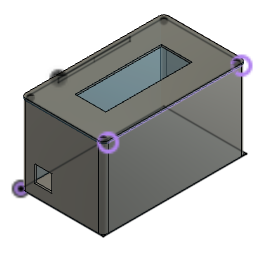
arduino_LED (Autodesk Fusion 360 design; units mm, degrees)
Autodesk Fusion 360 part; units mm, degrees
sketch "Base" plane through (0, 0, 0) normal (0, 1, 0) x (1, 0, 0) in component "Case"
  line L0 (0, 0) -> (68, 0)
  line L1 (68, 0) -> (68, 118)
  line L2 (68, 118) -> (0, 118)
  line L3 (0, 118) -> (0, 0)
  dimension "d6" = 68
  dimension "d7" = 118
  constraint horizontal L0
  constraint vertical L1
  constraint horizontal L2
  constraint vertical L3
  constraint coincident L0.start L3.end
  measures "d6" distance of L0.start L0.end
  measures "d7" distance of L0.start L2.end
extrude "Extrude1" add sketch "Base" along normal blind 65 makes body 1 in component "Case"
fillet "Fillet1" radius 4 4 edges at (68, 32.5, 0) (0, 32.5, 0) (68, 32.5, -118) (0, 32.5, -118) on bodies 1 in component "Case"
shell "Shell1" thickness 1.5 removed faces 1 at (22.6667, 65, -40.6667) on bodies 1 in component "Case"
sketch "Knob" plane through (1.5, 0, 0) normal (1, 0, 0) x (0, 0, -1) in component "Case"
  line L0 (114, 1.5) -> (114, 65)
  line L1 (114, 65) -> (4, 65)
  line L2 (4, 65) -> (4, 1.5)
  line L3 (4, 1.5) -> (114, 1.5)
  line L4 (29.5, 65) -> (88.5, 65)
  line L5 (88.5, 65) -> (88.5, 62)
  line L6 (88.5, 62) -> (29.5, 62)
  line L7 (29.5, 62) -> (29.5, 65)
  line L8 (59, 65) -> (59, 62) construction
  dimension "d12" = 59
  dimension "d13" = 3
  constraint horizontal L4
  constraint vertical L5
  constraint horizontal L6
  constraint vertical L7
  constraint coincident L1 L4.start
  constraint midpoint L1 L8.start
  constraint midpoint L6 L8.end
  constraint vertical L8
  measures "d12" distance of L5.end L6.end
  measures "d13" distance of L4.end L5.end
extrude "Extrude2" add sketch "Knob" along normal blind 6 draft -45 contours L1 L4 L5 L6 L7 bodies 1 in component "Case"
ref_plane "WorkPlane2" through (34, 32.5, -59) normal (-1, 0, 0) x (0, 0, 1) in component "Case"
mirror "Mirror1" about plane through (34, 32.5, -59) normal (-1, 0, 0) of "Extrude2" in component "Case"
sketch "Top" plane through (0, 65, 0) normal (0, 1, 0) x (-1, 0, 0) in component "Top Cover"
  line L0 (-68, -4) -> (-68, -114)
  arc A0 (-68, -114) -> (-64, -118) centre (-64, -114) ccw
  line L1 (-64, -118) -> (-4, -118)
  arc A1 (-4, -118) -> (0, -114) centre (-4, -114) ccw
  line L2 (0, -114) -> (0, -4)
  arc A2 (0, -4) -> (-4, 0) centre (-4, -4) ccw
  line L3 (-4, 0) -> (-64, 0)
  arc A3 (-64, 0) -> (-68, -4) centre (-64, -4) ccw
  line L4 (-66.5, -29.5) -> (-66.5, -4)
  arc A4 (-64, -1.5) -> (-66.5, -4) centre (-64, -4) ccw
  line L5 (-64, -1.5) -> (-4, -1.5)
  arc A5 (-1.5, -4) -> (-4, -1.5) centre (-4, -4) ccw
  line L6 (-1.5, -4) -> (-1.5, -29.5)
  line L7 (-1.5, -29.5) -> (-1.5, -88.5)
  line L8 (-1.5, -88.5) -> (-1.5, -114)
  arc A6 (-4, -116.5) -> (-1.5, -114) centre (-4, -114) ccw
  line L9 (-4, -116.5) -> (-64, -116.5)
  arc A7 (-66.5, -114) -> (-64, -116.5) centre (-64, -114) ccw
  line L10 (-66.5, -114) -> (-66.5, -88.5)
  line L11 (-66.5, -88.5) -> (-66.5, -29.5)
extrude "Extrude1'" add sketch "Top" along normal blind 1.5 separate body contours L0 A0 L1 A1 L2 A2 L3 A3 | L4 A4 L5 A5 L6 L7 L8 A6 L9 A7 L10 L11 makes body 2 in component "Top Cover"
sketch "Lip" plane through (0, 65, 0) normal (0, -1, 0) x (1, 0, 0) in component "Top Cover"
  arc A0 (68, -4) -> (64, 0) centre (64, -4) ccw
  line L0 (64, 0) -> (4, 0)
  arc A1 (4, 0) -> (0, -4) centre (4, -4) ccw
  line L1 (0, -4) -> (0, -114)
  arc A2 (0, -114) -> (4, -118) centre (4, -114) ccw
  line L2 (4, -118) -> (64, -118)
  arc A3 (64, -118) -> (68, -114) centre (64, -114) ccw
  line L3 (68, -114) -> (68, -4)
  line L4 (66.3, -114) -> (66.3, -4)
  arc A4 (66.3, -4) -> (64, -1.7) centre (64, -4) ccw
  line L5 (64, -1.7) -> (4, -1.7)
  arc A5 (4, -1.7) -> (1.7, -4) centre (4, -4) ccw
  line L6 (1.7, -4) -> (1.7, -114)
  arc A6 (1.7, -114) -> (4, -116.3) centre (4, -114) ccw
  line L7 (4, -116.3) -> (64, -116.3)
  arc A7 (64, -116.3) -> (66.3, -114) centre (64, -114) ccw
  line L8 (68, -4) -> (68, -114)
  dimension "d19" = 1.7
  dimension "d31" = 1.7
  measures "d31" distance of L4 L8
extrude "Extrude2'" add sketch "Lip" along normal blind 3 contours L4 A4 L5 A5 L6 A6 L7 A7 bodies 2 in component "Top Cover"
extrude "Extrude3" cut sketch "Knob" along normal blind 3 draft -45 from surface at 0.2 contours L1 L4 L5 L6 L7 bodies 2 in component "Top Cover"
ref_plane "WorkPlane2" through (34, 0, 0) normal (1, 0, 0) x (0, 1, 0) in component "Top Cover"
mirror "Mirror1'" about plane through (34, 0, 0) normal (1, 0, 0) of "Extrude3" in component "Top Cover"
shell "Shell1'" thickness 1.5 removed faces 1 at (44.7667, 62, -68.8333) on bodies 2 in component "Top Cover"
chamfer "Chamfer1" distance 0.6 angle 45 2 edges at (1.7, 62, -59) (66.3, 62, -59) on bodies 2 in component "Top Cover"
sketch "Sketch1" plane through (2.1865, 66.5, -5.8403) normal (0, 1, 0) x (-1, 0, 0)
  line L0 (-65.8135, 1.8403) -> (-65.8135, -108.1597)
  arc A0 (-65.8135, -108.1597) -> (-61.8135, -112.1597) centre (-61.8135, -108.1597) ccw
  line L1 (-61.8135, -112.1597) -> (-1.8135, -112.1597)
  arc A1 (-1.8135, -112.1597) -> (2.1865, -108.1597) centre (-1.8135, -108.1597) ccw
  line L2 (2.1865, -108.1597) -> (2.1865, 1.8403)
  arc A2 (2.1865, 1.8403) -> (-1.8135, 5.8403) centre (-1.8135, 1.8403) ccw
  line L3 (-1.8135, 5.8403) -> (-61.8135, 5.8403)
  arc A3 (-61.8135, 5.8403) -> (-65.8135, 1.8403) centre (-61.8135, 1.8403) ccw
  line L4 (-19.2135, -17.5597) -> (-44.4135, -17.5597)
  line L5 (-44.4135, -17.5597) -> (-44.4135, -88.7597)
  line L6 (-44.4135, -88.7597) -> (-19.2135, -88.7597)
  line L7 (-19.2135, -88.7597) -> (-19.2135, -17.5597)
  line L8 (2.1865, 5.8403) -> (-65.8135, 5.8403)
  line L9 (2.1865, -112.1597) -> (2.1865, 5.8403)
  dimension "d36" = 25.2
  dimension "d37" = 71.2
  dimension "d38" = 23.4
  dimension "d39" = 21.4
  constraint horizontal L4
  constraint vertical L5
  constraint horizontal L6
  constraint vertical L7
  measures "d36" distance of L4.start L4.end
  measures "d37" distance of L4.start L6.end
  measures "d38" distance of L4 L8
  measures "d39" distance of L7 L9
extrude "Extrude4" cut sketch "Sketch1" against normal blind 2 contours L4 L5 L6 L7 bodies 2 in component "Top Cover"
sketch "Sketch2" plane through (0, 0, 0) normal (0, 0, 1) x (1, 0, 0)
  line L0 (4, 65) -> (4, 0)
  line L1 (4, 0) -> (64, 0)
  line L2 (64, 0) -> (64, 65)
  line L3 (64, 65) -> (4, 65)
  line L4 (11.5, 23.5) -> (25.5, 23.5)
  line L5 (25.5, 23.5) -> (25.5, 9.5)
  line L6 (25.5, 9.5) -> (11.5, 9.5)
  line L7 (11.5, 9.5) -> (11.5, 23.5)
  line L8 (0, 65) -> (0, 0)
  line L9 (0, 0) -> (68, 0)
  dimension "d42" = 14
  dimension "d43" = 14
  dimension "d44" = 11.5
  dimension "d45" = 9.5
  constraint horizontal L4
  constraint vertical L5
  constraint horizontal L6
  constraint vertical L7
  measures "d42" distance of L4.start L4.end
  measures "d43" distance of L4.start L6.end
  measures "d44" distance of L7 L8
  measures "d45" distance of L6 L9
extrude "Extrude3'" cut sketch "Sketch2" against normal blind 2 contours L4 L5 L6 L7 bodies 1 in component "Case"
sketch "Sketch3" plane through (0, 0, 0) normal (-1, 0, 0) x (0, 0, 1)
  line L0 (-114, 65) -> (-114, 0)
  line L1 (-114, 0) -> (-4, 0)
  line L2 (-4, 0) -> (-4, 65)
  line L3 (-4, 65) -> (-114, 65)
  circle A0 centre (-59, 21.5) radius 3
  line L4 (0, 1.75) -> (0, 22.5)
  line L5 (-118, 0) -> (0, 0)
  dimension "d48" = 6
  dimension "d49" = 59
  dimension "d50" = 21.5
  measures "d48" diameter of A0
  measures "d49" distance of A0.centre L4
  measures "d50" distance of A0.centre L5
hole "Hole1" at (0, 21.5, -59) direction (1, 0, 0) diameter 6.5 depth 10 tip angle 180 bodies 1 in component "Case"
component "Enclosure" placed x (1, 0, 0) y (0, 1, 0) z (0, 0, 1) at (0, 0, 0)
component "Case" placed x (1, 0, 0) y (0, 1, 0) z (0, 0, 1) at (0, 0, 0) in component "Enclosure"
component "Top Cover" placed x (1, 0, 0) y (0, 1, 0) z (0, 0, 1) at (0, 0, 0) in component "Enclosure"
equation "Width = Width_internal + ( 2 * shell )"
equation "length = Length_internal + ( 2 * shell )"
equation "heigth = 65 mm"
equation "shell = 1.5 mm"
equation "gap = 0.2 mm"
equation "d6 = length"
equation "d7 = Width"
equation "d8 = heigth"
equation "d11 = shell"
equation "d12 = Width / 2"
equation "d13 = shell * 2"
equation "d17 = shell"
equation "d19 = shell + gap"
equation "d20 = shell * 2"
equation "d23 = shell * 2"
equation "d26 = shell"
equation "d31 = shell + gap"
equation "d33 = length / 2"
equation "Width_internal = 115 mm"
equation "Length_internal = 65 mm"
equation "d38 = Width / 2 - ( ( 71.2 / 2 ) * 1 mm )"
equation "d39 = ( length / 2 ) - ( ( 25.2 / 2 ) * 1 mm )"
equation "d44 = shell + 10 mm"
equation "d45 = shell + 8 mm"
equation "d49 = Width / 2"
equation "d50 = shell + 20 mm"
